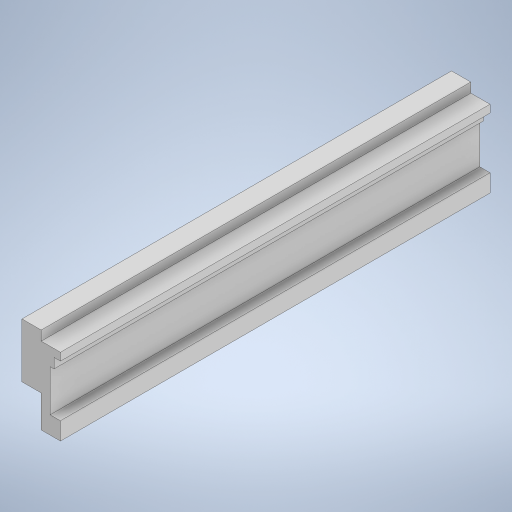
# Autodesk Inventor part: Diffuser
Saved by Autodesk Inventor 2023 (Build 270158000, 158)
## iProperties
Created: 2024-03-20
Part Number: Diffuser
Material: Generic
Document SubType Name: Modeling
Designer: noname
Density: 1 g/cm^3
Appearance: Default
Author: noname
Autodesk Inventor part; units mm, degrees
ref_plane "YZ Plane" through (0, 0, 0) normal (1, 0, 0) x (0, 1, 0)
ref_plane "XZ Plane" through (0, 0, 0) normal (0, 1, 0) x (-1, 0, 0)
ref_plane "XY Plane" through (0, 0, 0) normal (0, 0, 1) x (1, 0, 0)
sketch "Sketch1" plane through (0, 0, 0) normal (0, 0, 1) x (1, 0, 0)
  line L0 (0, 12) -> (0, 0)
  line L1 (0, 0) -> (-3, 0)
  line L2 (-3, 0) -> (-3, 5)
  line L3 (-3, 5) -> (-6, 5)
  line L4 (-6, 5) -> (-6, 13.5)
  line L5 (-6, 13.5) -> (-3, 13.5)
  line L6 (-3, 13.5) -> (-3, 12)
  line L7 (-3, 12) -> (0, 12)
  line L8 (0, 2.75) -> (-1.6, 2.75)
  line L9 (-1.6, 2.75) -> (-1.6, 9.25)
  line L10 (-1.6, 9.25) -> (0, 9.25)
  line L11 (0, 9.25) -> (0, 2.75)
  line L12 (0, 10.8) -> (-1, 10.8)
  line L13 (-1, 10.8) -> (-1, 9.25)
  line L14 (-1, 9.25) -> (0, 9.25)
  line L15 (0, 9.25) -> (0, 10.8)
  point P0 (-1.6, 6)
  point P1 (0, 9.25)
  point P2 (0, 9.25)
  dimension "d0" = 12
  dimension "d1" = 3
  dimension "d2" = 3
  dimension "d3" = 5
  dimension "d4" = 1.5
  dimension "d5" = 3
  dimension "d8" = 6
  dimension "d9" = 6.5
  dimension "d10" = 1.6
  dimension "d12" = 1.2
  dimension "d13" = 1
  constraints: 32 end point, 8 perpendicular, 4 parallel, 3 horizontal, 2 point on line, 1 midpoint, 1 vertical
  measures "d0" distance of L0.start L0.end
  measures "d1" distance between parallel lines of L0 L2
  measures "d2" distance between parallel lines of L2 L4
  measures "d3" distance between parallel lines of L1 L3
  measures "d4" distance between parallel lines of L7 L5
  measures "d5" distance between parallel lines of L0 L6
  measures "d8" distance from line of L1 point (-1.6, 6)
  measures "d9" distance between parallel lines of L8 L10
  measures "d10" distance between parallel lines of L11 L9
  measures "d12" distance between parallel lines of L7 L12
  measures "d13" distance between parallel lines of L15 L13
extrude "Extrusion1" add sketch "Sketch1" along normal blind 67 contours L0 L12 L13 L10 L9 L8 L1 L2 L3 L4 L5 L6 L7
body "Solid1"
